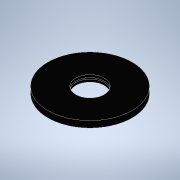
# Autodesk Inventor part: Push Rod Holder
Saved by Autodesk Inventor 2022 (Build 260153000, 153)
## iProperties
Created: 2023-01-26
Part Number: Push Rod Holder
Material: Generic
Document SubType Name: Modeling
Designer: ASUS
Density: 1 g/cm^3
Appearance: Rubber - Black
Author: ASUS
Autodesk Inventor part; units mm, degrees
ref_plane "YZ Plane" through (0, 0, 0) normal (1, 0, 0) x (0, 1, 0)
ref_plane "XZ Plane" through (0, 0, 0) normal (0, 1, 0) x (-1, 0, 0)
ref_plane "XY Plane" through (0, 0, 0) normal (0, 0, 1) x (1, 0, 0)
sketch "Sketch1" plane through (0, 0, 0) normal (0, 1, 0) x (-1, 0, 0)
  circle A0 centre (0, 0) radius 11
  circle A1 centre (0, 0) radius 32.5
  dimension "d0" = 22
  dimension "d1" = 65
  constraints: 2 centre point, 2 coincident
  measures "d0" diameter of A0
  measures "d1" diameter of A1
extrude "Extrusion1" add sketch "Sketch1" along normal blind 5
sketch "Sketch2" plane through (0, 0, 0) normal (1, 0, 0) x (0, 1, 0)
  line L0 (5, -11) -> (0, -11) projected
  arc A0 (2, -11) -> (3, -11) centre (2.5, -11) ccw
  line L1 (3, -11) -> (2, -11)
  line L2 (-1, 0) -> (6, 0) projected
  point P0 (0, 0)
  dimension "d4" = 1
  constraints: 2 end point, 2 point on circle, 2 point on line, 1 centre point, 1 horizontal, 1 midpoint
  measures "d4" diameter of A0
revolve "Revolution1" cut sketch "Sketch2" angle 360 about axis through (0, -10, 0) along (0, 1, 0)
body "Solid1"
